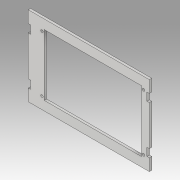
# Autodesk Inventor part: top_instrumentboard
Saved by Autodesk Inventor 2019.3 (Build 233278000, 278)
## iProperties
Created: 2019-05-28
Part Number: top_instrumentboard
Material: Generic
Document SubType Name: Modeling
Designer: Dave
Density: 1 g/cm^3
Appearance: Default
Author: Dave
Autodesk Inventor part; units mm, degrees
ref_plane "YZ Plane" through (0, 0, 0) normal (1, 0, 0) x (0, 1, 0)
ref_plane "XZ Plane" through (0, 0, 0) normal (0, 1, 0) x (-1, 0, 0)
ref_plane "XY Plane" through (0, 0, 0) normal (0, 0, 1) x (1, 0, 0)
sketch "Sketch1" plane through (0, 0, 0) normal (0, 0, 1) x (1, 0, 0)
  line L0 (0, 0) -> (152, 0)
  line L1 (152, 0) -> (152, 100)
  line L2 (152, 100) -> (0, 100)
  line L3 (0, 100) -> (0, 0)
  line L4 (20, 88.5) -> (142, 88.5)
  line L5 (142, 88.5) -> (142, 11.5)
  line L6 (142, 11.5) -> (20, 11.5)
  line L7 (20, 11.5) -> (20, 88.5)
  circle A0 centre (17.2, 85.3) radius 1.55
  circle A1 centre (17.2, 14.7) radius 1.55
  circle A2 centre (144.8, 85.3) radius 1.55
  circle A3 centre (144.8, 14.7) radius 1.55
  line L8 (0, 85) -> (3, 85)
  line L9 (3, 85) -> (3, 75)
  line L10 (3, 75) -> (0, 75)
  line L11 (0, 75) -> (0, 85)
  line L12 (0, 25) -> (3, 25)
  line L13 (3, 25) -> (3, 15)
  line L14 (3, 15) -> (0, 15)
  line L15 (0, 15) -> (0, 25)
  line L16 (152, 85) -> (149, 85)
  line L17 (149, 85) -> (149, 75)
  line L18 (149, 75) -> (152, 75)
  line L19 (152, 75) -> (152, 85)
  line L20 (152, 25) -> (149, 25)
  line L21 (149, 25) -> (149, 15)
  line L22 (149, 15) -> (152, 15)
  line L23 (152, 15) -> (152, 25)
  point P0 (81, 88.5)
  dimension "d0" = 122
  dimension "d1" = 77
  dimension "d3" = 10
  dimension "d5" = 11.5
  dimension "d6" = 3.1
  dimension "d7" = 127.6
  dimension "d8" = 63.8
  dimension "d9" = 70.6
  dimension "d10" = 3.2
  dimension "d11" = 3.2
  dimension "d14" = 100
  dimension "d15" = 11.5
  dimension "d16" = 152
  dimension "d17" = 20
  dimension "d18" = 3
  dimension "d19" = 10
  dimension "d20" = 15
  dimension "d21" = 15
  constraints: 48 end point, 12 parallel, 10 point on line, 6 horizontal, 6 perpendicular, 4 centre point, 3 equal radius, 2 collinear, 2 horizontal alignment, 2 vertical alignment, 1 midpoint
  measures "d0" distance of L4.start L4.end
  measures "d1" distance of L4.end L5.end
  measures "d3" distance between parallel lines of L1 L5
  measures "d5" distance between parallel lines of L6 L0
  measures "d6" diameter of A0
  measures "d7" distance of A2.centre A0.centre
  measures "d8" horizontal distance of A0.centre point (81, 88.5)
  measures "d9" distance of A3.centre A2.centre
  measures "d10" distance from line of L4 A0.centre
  measures "d11" distance from line of L6 A1.centre
  measures "d14" distance between parallel lines of L0 L2
  measures "d15" distance between parallel lines of L2 L4
  measures "d16" distance of L1.end L2.end
  measures "d17" distance between parallel lines of L3 L7
  measures "d18" distance of L8.start L8.end
  measures "d19" distance of L8.end L9.end
  measures "d20" distance between parallel lines of L2 L8
  measures "d21" distance between parallel lines of L0 L14
extrude "Extrusion1" add sketch "Sketch1" along normal blind 3 contours L3 L14 L13 L12 L10 L9 L8 L2 L1 L16 L17 L18 L20 L21 L22 L0
body "Solid1"
